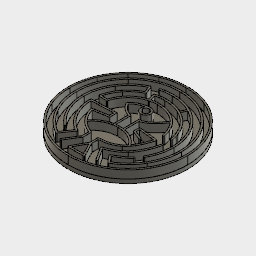
Maze 7_5 in (Autodesk Fusion 360 design; units mm, degrees)
Autodesk Fusion 360 part; units mm, degrees
sketch "Sketch5" plane through (0, 0, 0) normal (0, 1, 0) x (1, 0, 0)
  spline S0 degree 3 poles (-4.5755, 97.8232) (-27.1672, 97.8232) (-48.3865, 89.0258) (-64.3626, 73.0497) knots 0 0 0 0 1 1 1 1
  spline S1 degree 3 poles (-64.3626, 73.0497) (-80.3387, 57.0736) (-89.1009, 35.8895) (-89.1009, 13.2978) knots 0 0 0 0 1 1 1 1
  spline S2 degree 3 poles (-89.1009, 13.2978) (-89.1009, -1.7986) (-85.0541, -16.6134) (-77.4531, -29.5631) knots 0 0 0 0 1 1 1 1
  spline S3 degree 3 poles (-77.4531, -29.5631) (-70.0633, -42.1258) (-59.4713, -52.6123) (-46.8382, -59.9317) knots 0 0 0 0 1 1 1 1
  spline S4 degree 3 poles (-46.8382, -59.9317) (-46.2048, -60.2836) (-45.3954, -60.1077) (-44.9731, -59.5095) knots 0 0 0 0 1 1 1 1
  line L0 (-44.9731, -59.5095) -> (-31.9178, -40.9997)
  spline S5 degree 3 poles (-31.9178, -40.9997) (-31.4604, -40.3663) (-31.6363, -39.4866) (-32.2697, -39.0291) knots 0 0 0 0 1 1 1 1
  spline S6 degree 3 poles (-32.2697, -39.0291) (-32.3049, -38.9939) (-32.3753, -38.9939) (-32.4105, -38.9587) knots 0 0 0 0 1 1 1 1
  spline S7 degree 3 poles (-32.4105, -38.9587) (-50.2868, -29.0705) (-61.9345, -9.1884) (-62.3568, 11.9254) knots 0 0 0 0 1 1 1 1
  line L1 (-62.3568, 11.9254) -> (-27.8007, 13.2274)
  line L2 (-27.8007, 13.2274) -> (-27.8007, 6.3654)
  line L3 (-27.8007, 6.3654) -> (-50.7091, 2.389)
  spline S8 degree 3 poles (-50.7091, 2.389) (-51.5184, 2.2482) (-52.0463, 1.4037) (-51.8351, 0.6295) knots 0 0 0 0 1 1 1 1
  spline S9 degree 3 poles (-51.8351, 0.6295) (-47.7179, -14.7835) (-36.3869, -27.1351) (-21.4665, -32.6246) knots 0 0 0 0 1 1 1 1
  line L4 (-21.4665, -32.6246) -> (-21.4665, -43.6742)
  line L5 (-21.4665, -43.6742) -> (-34.2755, -64.0841)
  spline S10 degree 3 poles (-34.2755, -64.0841) (-34.6978, -64.7527) (-34.4867, -65.5973) (-33.8181, -66.0195) knots 0 0 0 0 1 1 1 1
  spline S11 degree 3 poles (-33.8181, -66.0195) (-33.5717, -66.1603) (-33.3254, -66.2307) (-33.0791, -66.2307) knots 0 0 0 0 1 1 1 1
  spline S12 degree 3 poles (-33.0791, -66.2307) (-32.6216, -66.2307) (-32.1642, -65.9843) (-31.8826, -65.5621) knots 0 0 0 0 1 1 1 1
  line L6 (-31.8826, -65.5621) -> (-18.6514, -44.4483)
  line L7 (-18.6514, -44.4483) -> (-18.6514, -31.6041)
  spline S13 degree 3 poles (-18.6514, -31.6041) (-18.6514, -31.0059) (-19.0384, -30.478) (-19.6015, -30.2669) knots 0 0 0 0 1 1 1 1
  spline S14 degree 3 poles (-19.6015, -30.2669) (-26.3227, -27.9444) (-32.2697, -24.1791) (-37.1611, -19.323) knots 0 0 0 0 1 1 1 1
  spline S15 degree 3 poles (-37.1611, -19.323) (-29.3842, -9.2235) (-17.279, -3.2061) (-4.5756, -3.2061) knots 0 0 0 0 1 1 1 1
  spline S16 degree 3 poles (-4.5756, -3.2061) (9.1484, -3.2061) (20.6906, -8.8717) (28.0804, -19.2526) knots 0 0 0 0 1 1 1 1
  spline S17 degree 3 poles (28.0804, -19.2526) (26.6024, -21.0472) (25.0541, -22.5604) (23.5057, -23.792) knots 0 0 0 0 1 1 1 1
  spline S18 degree 3 poles (23.5057, -23.792) (16.0104, -29.7743) (6.5796, -32.8006) (-4.5755, -32.8006) knots 0 0 0 0 1 1 1 1
  spline S19 degree 3 poles (-4.5755, -32.8006) (-5.3497, -32.8006) (-5.9831, -33.434) (-5.9831, -34.2082) knots 0 0 0 0 1 1 1 1
  line L8 (-5.9831, -34.2082) -> (-5.9831, -45.8207)
  line L9 (-5.9831, -45.8207) -> (-18.1235, -67.9198)
  spline S20 degree 3 poles (-18.1235, -67.9198) (-18.3698, -68.342) (-18.3698, -68.8699) (-18.0883, -69.3274) knots 0 0 0 0 1 1 1 1
  spline S21 degree 3 poles (-18.0883, -69.3274) (-17.842, -69.7496) (-17.3845, -70.0311) (-16.8919, -70.0311) knots 0 0 0 0 1 1 1 1
  line L10 (-16.8919, -70.0311) -> (7.0371, -70.0311)
  spline S22 degree 3 poles (7.0371, -70.0311) (7.5297, -70.0311) (7.9872, -69.7848) (8.2335, -69.3625) knots 0 0 0 0 1 1 1 1
  spline S23 degree 3 poles (8.2335, -69.3625) (8.4798, -68.9403) (8.515, -68.4124) (8.2687, -67.9901) knots 0 0 0 0 1 1 1 1
  line L11 (8.2687, -67.9901) -> (-3.1679, -45.8207)
  line L12 (-3.1679, -45.8207) -> (-3.1679, -35.5806)
  spline S24 degree 3 poles (-3.1679, -35.5806) (8.0224, -35.3342) (17.5587, -32.132) (25.2653, -26.009) knots 0 0 0 0 1 1 1 1
  spline S25 degree 3 poles (25.2653, -26.009) (33.2885, -19.6397) (40.7487, -5.9861) (44.3028, 8.7583) knots 0 0 0 0 1 1 1 1
  spline S26 degree 3 poles (44.3028, 8.7583) (44.4084, 9.1454) (44.3028, 9.5677) (44.0917, 9.8844) knots 0 0 0 0 1 1 1 1
  spline S27 degree 3 poles (44.0917, 9.8844) (43.8454, 10.2011) (43.4935, 10.4474) (43.1064, 10.4826) knots 0 0 0 0 1 1 1 1
  line L13 (43.1064, 10.4826) -> (14.6028, 13.6497)
  spline S28 degree 3 poles (14.6028, 13.6497) (14.2157, 13.6849) (13.7935, 13.5793) (13.5119, 13.2978) knots 0 0 0 0 1 1 1 1
  spline S29 degree 3 poles (13.5119, 13.2978) (13.2304, 13.0163) (13.0545, 12.6644) (13.0545, 12.2421) knots 0 0 0 0 1 1 1 1
  line L14 (13.0545, 12.2421) -> (13.0545, 4.4709)
  spline S30 degree 3 poles (13.0545, 4.4709) (13.0545, 3.943) (13.3712, 3.4152) (13.8638, 3.2041) knots 0 0 0 0 1 1 1 1
  line L15 (13.8638, 3.2041) -> (27.7716, -2.4085)
  spline S31 degree 3 poles (27.7716, -2.4085) (28.4754, -2.7252) (29.3199, -2.4436) (29.6366, -1.7399) knots 0 0 0 0 1 1 1 1
  spline S32 degree 3 poles (29.6366, -1.7399) (29.9533, -1.0361) (29.6718, -0.1915) (28.968, 0.1252) knots 0 0 0 0 1 1 1 1
  line L16 (28.968, 0.1252) -> (15.8345, 5.3506)
  line L17 (15.8345, 5.3506) -> (15.8345, 10.6586)
  line L18 (15.8345, 10.6586) -> (41.171, 7.8434)
  spline S33 degree 3 poles (41.171, 7.8434) (38.7077, -1.6578) (34.5905, -10.5256) (29.8751, -16.9653) knots 0 0 0 0 1 1 1 1
  spline S34 degree 3 poles (29.8751, -16.9653) (23.6114, -8.5549) (14.7436, -3.1358) (4.2219, -1.2003) knots 0 0 0 0 1 1 1 1
  line L19 (4.2219, -1.2003) -> (4.2219, 21.6377)
  spline S35 degree 3 poles (4.2219, 21.6377) (15.4474, 24.1714) (24.5967, 35.4672) (30.79, 44.5109) knots 0 0 0 0 1 1 1 1
  spline S36 degree 3 poles (30.79, 44.5109) (34.133, 40.816) (36.8074, 36.5581) (38.6373, 31.8075) knots 0 0 0 0 1 1 1 1
  spline S37 degree 3 poles (38.6373, 31.8075) (40.5023, 27.0217) (40.5023, 27.0217) (41.4876, 21.9544) knots 0 0 0 0 1 1 1 1
  line L20 (41.4876, 21.9544) -> (41.5228, 21.8137)
  spline S38 degree 3 poles (41.5228, 21.8137) (41.6636, 21.1451) (42.2266, 20.6876) (42.8952, 20.6876) knots 0 0 0 0 1 1 1 1
  spline S39 degree 3 poles (42.8952, 20.6876) (43.0008, 20.6876) (43.0712, 20.6876) (43.1767, 20.7228) knots 0 0 0 0 1 1 1 1
  spline S40 degree 3 poles (43.1767, 20.7228) (43.9509, 20.8635) (44.4436, 21.6025) (44.2676, 22.3767) knots 0 0 0 0 1 1 1 1
  line L21 (44.2676, 22.3767) -> (44.2324, 22.5174)
  spline S41 degree 3 poles (44.2324, 22.5174) (43.1767, 27.7607) (43.1416, 27.8663) (41.2413, 32.828) knots 0 0 0 0 1 1 1 1
  spline S42 degree 3 poles (41.2413, 32.828) (34.3442, 50.6691) (16.3623, 62.2113) (-4.5755, 62.2113) knots 0 0 0 0 1 1 1 1
  spline S43 degree 3 poles (-4.5755, 62.2113) (-8.4815, 62.2113) (-12.282, 61.7538) (-15.9417, 60.8741) knots 0 0 0 0 1 1 1 1
  line L22 (-15.9417, 60.8741) -> (-18.3346, 69.39)
  spline S44 degree 3 poles (-18.3346, 69.39) (-13.7952, 70.5161) (-9.115, 71.0791) (-4.3996, 71.0791) knots 0 0 0 0 1 1 1 1
  spline S45 degree 3 poles (-4.3996, 71.0791) (4.5034, 71.0791) (13.0193, 69.214) (20.9018, 65.5895) knots 0 0 0 0 1 1 1 1
  spline S46 degree 3 poles (20.9018, 65.5895) (34.9424, 59.0794) (45.3937, 47.6428) (50.3906, 33.3207) knots 0 0 0 0 1 1 1 1
  spline S47 degree 3 poles (50.3906, 33.3207) (50.9537, 31.7019) (51.3407, 30.6463) (51.6223, 29.8721) knots 0 0 0 0 1 1 1 1
  spline S48 degree 3 poles (51.6223, 29.8721) (52.3964, 27.7959) (52.502, 27.5496) (53.5225, 22.5175) knots 0 0 0 0 1 1 1 1
  spline S49 degree 3 poles (53.5225, 22.5175) (53.6633, 21.8489) (54.2263, 21.3914) (54.8949, 21.3914) knots 0 0 0 0 1 1 1 1
  spline S50 degree 3 poles (54.8949, 21.3914) (55.0005, 21.3914) (55.0709, 21.3914) (55.1764, 21.4266) knots 0 0 0 0 1 1 1 1
  spline S51 degree 3 poles (55.1764, 21.4266) (55.9506, 21.5673) (56.4432, 22.3063) (56.2673, 23.0805) knots 0 0 0 0 1 1 1 1
  spline S52 degree 3 poles (56.2673, 23.0805) (55.2116, 28.3238) (55.0708, 28.7108) (54.2615, 30.8926) knots 0 0 0 0 1 1 1 1
  spline S53 degree 3 poles (54.2615, 30.8926) (53.9448, 31.702) (53.5929, 32.6873) (53.0298, 34.2708) knots 0 0 0 0 1 1 1 1
  spline S54 degree 3 poles (53.0298, 34.2708) (48.1737, 48.2762) (38.2854, 59.6777) (25.0541, 66.7156) knots 0 0 0 0 1 1 1 1
  line L23 (25.0541, 66.7156) -> (28.7842, 74.7036)
  spline S55 degree 3 poles (28.7842, 74.7036) (51.3407, 62.4225) (65.2758, 39.0566) (65.2758, 13.333) knots 0 0 0 0 1 1 1 1
  spline S56 degree 3 poles (65.2758, 13.333) (65.2758, 0.9463) (62.0032, -11.1941) (55.7746, -21.8214) knots 0 0 0 0 1 1 1 1
  spline S57 degree 3 poles (55.7746, -21.8214) (55.3876, -22.49) (55.5987, -23.3697) (56.2673, -23.7568) knots 0 0 0 0 1 1 1 1
  spline S58 degree 3 poles (56.2673, -23.7568) (56.4784, -23.8976) (56.7248, -23.9328) (56.9711, -23.9328) knots 0 0 0 0 1 1 1 1
  spline S59 degree 3 poles (56.9711, -23.9328) (57.4637, -23.9328) (57.9212, -23.6864) (58.2027, -23.229) knots 0 0 0 0 1 1 1 1
  spline S60 degree 3 poles (58.2027, -23.229) (64.6424, -12.1794) (68.0558, 0.4888) (68.0558, 13.3682) knots 0 0 0 0 1 1 1 1
  spline S61 degree 3 poles (68.0558, 13.3682) (68.0558, 40.6401) (52.9947, 65.3784) (28.749, 77.9411) knots 0 0 0 0 1 1 1 1
  spline S62 degree 3 poles (28.749, 77.9411) (18.5089, 83.2547) (6.9667, 86.0347) (-4.6107, 86.0347) knots 0 0 0 0 1 1 1 1
  spline S63 degree 3 poles (-4.6107, 86.0347) (-10.98, 86.0347) (-17.3141, 85.1901) (-23.4371, 83.5714) knots 0 0 0 0 1 1 1 1
  spline S64 degree 3 poles (-23.4371, 83.5714) (-24.1761, 83.3603) (-24.6336, 82.5861) (-24.4224, 81.8471) knots 0 0 0 0 1 1 1 1
  spline S65 degree 3 poles (-24.4224, 81.8471) (-24.2113, 81.1081) (-23.4371, 80.6507) (-22.6981, 80.8618) knots 0 0 0 0 1 1 1 1
  spline S66 degree 3 poles (-22.6981, 80.8618) (-16.8215, 82.4453) (-10.7337, 83.2195) (-4.6107, 83.2195) knots 0 0 0 0 1 1 1 1
  spline S67 degree 3 poles (-4.6107, 83.2195) (6.2277, 83.2195) (16.6086, 80.7914) (26.2506, 76.0409) knots 0 0 0 0 1 1 1 1
  line L24 (26.2506, 76.0409) -> (22.5205, 67.9472)
  spline S68 degree 3 poles (22.5205, 67.9472) (22.3797, 68.0176) (22.239, 68.088) (22.063, 68.1583) knots 0 0 0 0 1 1 1 1
  spline S69 degree 3 poles (22.063, 68.1583) (13.8286, 71.994) (4.8905, 73.9294) (-4.4347, 73.9294) knots 0 0 0 0 1 1 1 1
  spline S70 degree 3 poles (-4.4347, 73.9294) (-9.8891, 73.9294) (-15.2731, 73.2256) (-20.4812, 71.7829) knots 0 0 0 0 1 1 1 1
  spline S71 degree 3 poles (-20.4812, 71.7829) (-21.2202, 71.5717) (-21.6776, 70.7976) (-21.4665, 70.0586) knots 0 0 0 0 1 1 1 1
  spline S72 degree 3 poles (-21.4665, 70.0586) (-21.4665, 70.0234) (-21.4665, 70.0234) (-21.4313, 69.9882) knots 0 0 0 0 1 1 1 1
  spline S73 degree 3 poles (-21.4313, 69.9882) (-21.4313, 69.953) (-21.4313, 69.953) (-21.4313, 69.9178) knots 0 0 0 0 1 1 1 1
  line L25 (-21.4313, 69.9178) -> (-18.6865, 60.1351)
  spline S74 degree 3 poles (-18.6865, 60.1351) (-34.2403, 55.4549) (-46.8382, 43.1737) (-51.5536, 27.0569) knots 0 0 0 0 1 1 1 1
  line L26 (-51.5536, 27.0569) -> (-60.5973, 27.5496)
  spline S75 degree 3 poles (-60.5973, 27.5496) (-58.5915, 35.432) (-54.8614, 42.9274) (-49.7589, 49.2967) knots 0 0 0 0 1 1 1 1
  spline S76 degree 3 poles (-49.7589, 49.2967) (-44.3749, 56.0179) (-37.4426, 61.5779) (-29.7009, 65.3432) knots 0 0 0 0 1 1 1 1
  spline S77 degree 3 poles (-29.7009, 65.3432) (-29.0322, 65.6599) (-28.7156, 66.434) (-28.9971, 67.1026) knots 0 0 0 0 1 1 1 1
  line L27 (-28.9971, 67.1026) -> (-33.3958, 78.3985)
  spline S78 degree 3 poles (-33.3958, 78.3985) (-33.5366, 78.7504) (-33.8181, 79.0319) (-34.17, 79.2079) knots 0 0 0 0 1 1 1 1
  spline S79 degree 3 poles (-34.17, 79.2079) (-34.5219, 79.3486) (-34.9441, 79.3486) (-35.296, 79.1727) knots 0 0 0 0 1 1 1 1
  spline S80 degree 3 poles (-35.296, 79.1727) (-47.6476, 73.4016) (-58.0989, 64.2875) (-65.5591, 52.8157) knots 0 0 0 0 1 1 1 1
  spline S81 degree 3 poles (-65.5591, 52.8157) (-73.1952, 41.0624) (-77.242, 27.3736) (-77.242, 13.2978) knots 0 0 0 0 1 1 1 1
  spline S82 degree 3 poles (-77.242, 13.2978) (-77.242, -8.2382) (-67.776, -28.5074) (-51.2721, -42.3721) knots 0 0 0 0 1 1 1 1
  spline S83 degree 3 poles (-51.2721, -42.3721) (-51.0258, -42.5833) (-50.6739, -42.6889) (-50.3572, -42.6889) knots 0 0 0 0 1 1 1 1
  spline S84 degree 3 poles (-50.3572, -42.6889) (-49.9701, -42.6889) (-49.5478, -42.5129) (-49.2663, -42.1962) knots 0 0 0 0 1 1 1 1
  spline S85 degree 3 poles (-49.2663, -42.1962) (-48.7736, -41.598) (-48.844, -40.7182) (-49.4422, -40.2256) knots 0 0 0 0 1 1 1 1
  spline S86 degree 3 poles (-49.4422, -40.2256) (-65.3128, -26.8887) (-74.3917, -7.3937) (-74.3917, 13.2978) knots 0 0 0 0 1 1 1 1
  spline S87 degree 3 poles (-74.3917, 13.2978) (-74.3917, 26.8458) (-70.5208, 39.9715) (-63.1662, 51.3025) knots 0 0 0 0 1 1 1 1
  spline S88 degree 3 poles (-63.1662, 51.3025) (-56.269, 61.8946) (-46.6975, 70.4105) (-35.4368, 75.9704) knots 0 0 0 0 1 1 1 1
  line L28 (-35.4368, 75.9704) -> (-32.0234, 67.2786)
  spline S89 degree 3 poles (-32.0234, 67.2786) (-39.6595, 63.3726) (-46.5215, 57.7774) (-51.8703, 51.0562) knots 0 0 0 0 1 1 1 1
  spline S90 degree 3 poles (-51.8703, 51.0562) (-57.571, 43.9127) (-61.653, 35.432) (-63.6588, 26.5291) knots 0 0 0 0 1 1 1 1
  spline S91 degree 3 poles (-63.6588, 26.5291) (-63.6588, 26.4587) (-63.694, 26.3883) (-63.694, 26.2827) knots 0 0 0 0 1 1 1 1
  spline S92 degree 3 poles (-63.694, 26.2827) (-63.7292, 25.5086) (-63.131, 24.84) (-62.3568, 24.8048) knots 0 0 0 0 1 1 1 1
  line L29 (-62.3568, 24.8048) -> (-50.4979, 24.1714)
  spline S93 degree 3 poles (-50.4979, 24.1714) (-50.0053, 24.1362) (-49.5478, 24.3825) (-49.2663, 24.8048) knots 0 0 0 0 1 1 1 1
  spline S94 degree 3 poles (-49.2663, 24.8048) (-49.1607, 24.9455) (-49.0904, 25.0863) (-49.0552, 25.2622) knots 0 0 0 0 1 1 1 1
  spline S95 degree 3 poles (-49.0552, 25.2622) (-44.7972, 41.2031) (-32.4105, 53.3083) (-17.0678, 57.6366) knots 0 0 0 0 1 1 1 1
  spline S96 degree 3 poles (-17.0678, 57.6366) (-16.9974, 57.6366) (-16.9271, 57.6014) (-16.8567, 57.6014) knots 0 0 0 0 1 1 1 1
  spline S97 degree 3 poles (-16.8567, 57.6014) (-16.7159, 57.6014) (-16.6104, 57.6014) (-16.4696, 57.6718) knots 0 0 0 0 1 1 1 1
  spline S98 degree 3 poles (-16.4696, 57.6718) (-16.2585, 57.7422) (-16.1177, 57.8126) (-15.9418, 57.9533) knots 0 0 0 0 1 1 1 1
  spline S99 degree 3 poles (-15.9418, 57.9533) (-12.2821, 58.9035) (-8.4464, 59.3961) (-4.5052, 59.3961) knots 0 0 0 0 1 1 1 1
  spline S100 degree 3 poles (-4.5052, 59.3961) (8.5854, 59.3961) (20.4443, 54.6455) (28.8546, 46.5519) knots 0 0 0 0 1 1 1 1
  spline S101 degree 3 poles (28.8546, 46.5519) (22.7316, 37.5434) (13.5471, 26.0012) (2.6383, 24.1713) knots 0 0 0 0 1 1 1 1
  spline S102 degree 3 poles (2.6383, 24.1713) (1.9697, 24.0658) (1.4771, 23.4676) (1.4771, 22.799) knots 0 0 0 0 1 1 1 1
  line L30 (1.4771, 22.799) -> (1.4771, -0.7781)
  spline S103 degree 3 poles (1.4771, -0.7781) (-0.4584, -0.5317) (-2.4642, -0.4262) (-4.5052, -0.4262) knots 0 0 0 0 1 1 1 1
  spline S104 degree 3 poles (-4.5052, -0.4262) (-6.4054, -0.4262) (-8.2705, -0.5669) (-10.1355, -0.8133) knots 0 0 0 0 1 1 1 1
  line L31 (-10.1355, -0.8133) -> (-10.1355, 22.7286)
  spline S105 degree 3 poles (-10.1355, 22.7286) (-10.1003, 23.3972) (-10.5578, 24.0306) (-11.2264, 24.1714) knots 0 0 0 0 1 1 1 1
  spline S106 degree 3 poles (-11.2264, 24.1714) (-18.1939, 25.6845) (-23.8242, 29.9776) (-28.4341, 37.2619) knots 0 0 0 0 1 1 1 1
  spline S107 degree 3 poles (-28.4341, 37.2619) (-23.6835, 41.9773) (-17.8068, 45.1443) (-11.3671, 46.4464) knots 0 0 0 0 1 1 1 1
  spline S108 degree 3 poles (-11.3671, 46.4464) (-12.3524, 45.074) (-12.9507, 43.4201) (-12.9507, 41.5902) knots 0 0 0 0 1 1 1 1
  spline S109 degree 3 poles (-12.9507, 41.5902) (-12.9507, 37.0156) (-9.2558, 33.3207) (-4.6811, 33.3207) knots 0 0 0 0 1 1 1 1
  spline S110 degree 3 poles (-4.6811, 33.3207) (-0.1065, 33.3207) (3.5884, 37.0156) (3.5884, 41.5902) knots 0 0 0 0 1 1 1 1
  spline S111 degree 3 poles (3.5884, 41.5902) (3.5884, 46.0945) (-0.0361, 49.7542) (-4.5052, 49.8598) knots 0 0 0 0 1 1 1 1
  line L32 (-4.5052, 49.8598) -> (-4.5052, 49.9653)
  spline S112 degree 3 poles (-4.5052, 49.9653) (-14.675, 49.9653) (-24.141, 45.8833) (-31.1437, 38.5287) knots 0 0 0 0 1 1 1 1
  spline S113 degree 3 poles (-31.1437, 38.5287) (-31.1789, 38.4935) (-31.1789, 38.4935) (-31.2141, 38.4583) knots 0 0 0 0 1 1 1 1
  spline S114 degree 3 poles (-31.2141, 38.4583) (-31.6363, 38.0009) (-31.7419, 37.3323) (-31.39, 36.7692) knots 0 0 0 0 1 1 1 1
  spline S115 degree 3 poles (-31.39, 36.7692) (-26.4987, 28.6404) (-20.4461, 23.7139) (-12.9155, 21.7433) knots 0 0 0 0 1 1 1 1
  line L33 (-12.9155, 21.7433) -> (-12.9155, -1.2707)
  spline S116 degree 3 poles (-12.9155, -1.2707) (-23.1205, -3.3117) (-32.4457, -8.942) (-38.991, -17.282) knots 0 0 0 0 1 1 1 1
  spline S117 degree 3 poles (-38.991, -17.282) (-43.3193, -12.3906) (-46.6271, -6.5491) (-48.5625, -0.1095) knots 0 0 0 0 1 1 1 1
  line L34 (-48.5625, -0.1095) -> (-24.8447, 4.0429)
  line L35 (-24.8447, 4.0429) -> (-24.8447, 16.1833)
  line L36 (-24.8447, 16.1833) -> (-63.7644, 14.7054)
  spline S118 degree 3 poles (-63.7644, 14.7054) (-64.5386, 14.6702) (-65.1368, 14.0368) (-65.1016, 13.2626) knots 0 0 0 0 1 1 1 1
  spline S119 degree 3 poles (-65.1016, 13.2626) (-65.1016, 13.2274) (-65.1016, 13.1922) (-65.1016, 13.157) knots 0 0 0 0 1 1 1 1
  line L37 (-65.1016, 13.157) -> (-65.2072, 13.157)
  spline S120 degree 3 poles (-65.2072, 13.157) (-65.2072, -8.8716) (-53.4538, -29.8094) (-35.1201, -40.6126) knots 0 0 0 0 1 1 1 1
  line L38 (-35.1201, -40.6126) -> (-46.5567, -56.7998)
  spline S121 degree 3 poles (-46.5567, -56.7998) (-58.2748, -49.7619) (-68.0927, -39.8737) (-75.025, -28.0852) knots 0 0 0 0 1 1 1 1
  spline S122 degree 3 poles (-75.025, -28.0852) (-82.3797, -15.5929) (-86.2857, -1.2355) (-86.2857, 13.3682) knots 0 0 0 0 1 1 1 1
  spline S123 degree 3 poles (-86.2857, 13.3682) (-86.2857, 35.1857) (-77.7698, 55.7364) (-62.3568, 71.1495) knots 0 0 0 0 1 1 1 1
  spline S124 degree 3 poles (-62.3568, 71.1495) (-46.9438, 86.5625) (-26.393, 95.0784) (-4.5755, 95.0784) knots 0 0 0 0 1 1 1 1
  spline S125 degree 3 poles (-4.5755, 95.0784) (17.242, 95.0784) (37.7928, 86.5625) (53.2058, 71.1495) knots 0 0 0 0 1 1 1 1
  spline S126 degree 3 poles (53.2058, 71.1495) (68.6188, 55.7364) (77.1347, 35.1857) (77.1347, 13.3682) knots 0 0 0 0 1 1 1 1
  spline S127 degree 3 poles (77.1347, 13.3682) (77.1347, -1.2355) (73.2287, -15.5577) (65.874, -28.0852) knots 0 0 0 0 1 1 1 1
  spline S128 degree 3 poles (65.874, -28.0852) (58.9065, -39.9088) (49.0534, -49.7971) (37.3001, -56.8351) knots 0 0 0 0 1 1 1 1
  line L39 (37.3001, -56.8351) -> (30.2974, -48.6007)
  spline S129 degree 3 poles (30.2974, -48.6007) (37.3705, -44.5187) (45.9567, -39.4514) (51.0592, -33.3636) knots 0 0 0 0 1 1 1 1
  spline S130 degree 3 poles (51.0592, -33.3636) (51.5519, -32.7654) (51.4815, -31.8856) (50.8833, -31.393) knots 0 0 0 0 1 1 1 1
  spline S131 degree 3 poles (50.8833, -31.393) (50.285, -30.9003) (49.4053, -30.9707) (48.9127, -31.5689) knots 0 0 0 0 1 1 1 1
  spline S132 degree 3 poles (48.9127, -31.5689) (43.9509, -37.4808) (35.2239, -42.5129) (28.2564, -46.5597) knots 0 0 0 0 1 1 1 1
  line L40 (28.2564, -46.5597) -> (27.447, -47.0171)
  spline S133 degree 3 poles (27.447, -47.0171) (27.0951, -47.2283) (26.8488, -47.5802) (26.7784, -48.0025) knots 0 0 0 0 1 1 1 1
  spline S134 degree 3 poles (26.7784, -48.0025) (26.708, -48.4247) (26.8136, -48.847) (27.0951, -49.1637) knots 0 0 0 0 1 1 1 1
  line L41 (27.0951, -49.1637) -> (35.9277, -59.5798)
  spline S135 degree 3 poles (35.9277, -59.5798) (36.2092, -59.8965) (36.5963, -60.0725) (37.0186, -60.0725) knots 0 0 0 0 1 1 1 1
  spline S136 degree 3 poles (37.0186, -60.0725) (37.2649, -60.0725) (37.5112, -60.0021) (37.7224, -59.8965) knots 0 0 0 0 1 1 1 1
  spline S137 degree 3 poles (37.7224, -59.8965) (50.3554, -52.6123) (60.9123, -42.0906) (68.3373, -29.5279) knots 0 0 0 0 1 1 1 1
  spline S138 degree 3 poles (68.3373, -29.5279) (75.9734, -16.5782) (79.985, -1.7633) (79.985, 13.333) knots 0 0 0 0 1 1 1 1
  spline S139 degree 3 poles (79.985, 13.333) (79.985, 35.9247) (71.1876, 57.144) (55.2116, 73.1201) knots 0 0 0 0 1 1 1 1
  spline S140 degree 3 poles (55.2116, 73.1201) (39.2355, 89.061) (18.0162, 97.8232) (-4.5755, 97.8232) knots 0 0 0 0 1 1 1 1
  line L42 (-14.5342, -67.1808) -> (-4.6107, -49.1637)
  line L43 (-4.6107, -49.1637) -> (4.7497, -67.1808)
  line L44 (4.7497, -67.1808) -> (-14.5342, -67.1808)
  spline S141 degree 3 poles (0.7029, 41.6254) (0.7029, 38.6343) (-1.7603, 36.171) (-4.7515, 36.171) knots 0 0 0 0 1 1 1 1
  spline S142 degree 3 poles (-4.7515, 36.171) (-7.7426, 36.171) (-10.2058, 38.6343) (-10.2058, 41.6254) knots 0 0 0 0 1 1 1 1
  spline S143 degree 3 poles (-10.2058, 41.6254) (-10.2058, 44.6165) (-7.7426, 47.0798) (-4.7515, 47.0798) knots 0 0 0 0 1 1 1 1
  spline S144 degree 3 poles (-4.7515, 47.0798) (-1.7603, 47.0798) (0.7029, 44.6165) (0.7029, 41.6254) knots 0 0 0 0 1 1 1 1
  spline S145 degree 3 poles (13.0193, -45.1169) (22.3797, -42.3018) (31.1067, -36.9529) (38.3206, -29.5983) knots 0 0 0 0 1 1 1 1
  spline S146 degree 3 poles (38.3206, -29.5983) (47.2236, -20.5194) (53.8744, -3.8747) (56.2673, 7.7378) knots 0 0 0 0 1 1 1 1
  spline S147 degree 3 poles (56.2673, 7.7378) (56.4081, 8.512) (55.9506, 9.251) (55.1764, 9.3917) knots 0 0 0 0 1 1 1 1
  spline S148 degree 3 poles (55.1764, 9.3917) (54.4022, 9.5325) (53.6633, 9.075) (53.5225, 8.3009) knots 0 0 0 0 1 1 1 1
  spline S149 degree 3 poles (53.5225, 8.3009) (50.2147, -7.7104) (42.297, -21.5751) (36.35, -27.6277) knots 0 0 0 0 1 1 1 1
  spline S150 degree 3 poles (36.35, -27.6277) (29.0306, -35.0879) (20.0924, -40.3663) (10.5208, -42.9352) knots 0 0 0 0 1 1 1 1
  spline S151 degree 3 poles (10.5208, -42.9352) (9.7819, -43.1463) (9.3244, -43.9205) (9.5355, -44.6595) knots 0 0 0 0 1 1 1 1
  spline S152 degree 3 poles (9.5355, -44.6595) (9.5355, -44.6946) (9.5355, -44.6946) (9.5707, -44.7298) knots 0 0 0 0 1 1 1 1
  spline S153 degree 3 poles (9.5707, -44.7298) (9.6059, -44.9058) (9.6763, -45.0466) (9.7467, -45.1873) knots 0 0 0 0 1 1 1 1
  line L45 (9.7467, -45.1873) -> (22.7668, -65.5973)
  spline S154 degree 3 poles (22.7668, -65.5973) (23.0483, -66.0195) (23.5058, -66.2307) (23.9633, -66.2307) knots 0 0 0 0 1 1 1 1
  spline S155 degree 3 poles (23.9633, -66.2307) (24.2096, -66.2307) (24.4911, -66.1603) (24.7022, -66.0195) knots 0 0 0 0 1 1 1 1
  spline S156 degree 3 poles (24.7022, -66.0195) (25.3708, -65.5973) (25.5468, -64.7175) (25.1245, -64.0841) knots 0 0 0 0 1 1 1 1
  line L46 (25.1245, -64.0841) -> (13.0193, -45.1169)
  spline S157 degree 3 poles (-4.9274, 108.3097) (-57.3951, 108.3097) (-99.9393, 65.7655) (-99.9393, 13.2978) knots 0 0 0 0 1 1 1 1
  spline S158 degree 3 poles (-99.9393, 13.2978) (-99.9393, -39.1699) (-57.3951, -81.7141) (-4.9274, -81.7141) knots 0 0 0 0 1 1 1 1
  spline S159 degree 3 poles (-4.9274, -81.7141) (47.5403, -81.7141) (90.0845, -39.1699) (90.0845, 13.2978) knots 0 0 0 0 1 1 1 1
  spline S160 degree 3 poles (90.0845, 13.2978) (90.0845, 65.7654) (47.5403, 108.3097) (-4.9274, 108.3097) knots 0 0 0 0 1 1 1 1
  spline S161 degree 3 poles (60.2789, -51.9085) (51.7982, -60.3892) (41.9451, -67.04) (30.966, -71.6851) knots 0 0 0 0 1 1 1 1
  spline S162 degree 3 poles (30.966, -71.6851) (19.5997, -76.506) (7.5297, -78.9341) (-4.9274, -78.9341) knots 0 0 0 0 1 1 1 1
  spline S163 degree 3 poles (-4.9274, -78.9341) (-17.3845, -78.9341) (-29.4545, -76.506) (-40.8208, -71.6851) knots 0 0 0 0 1 1 1 1
  spline S164 degree 3 poles (-40.8208, -71.6851) (-51.7999, -67.04) (-61.653, -60.3892) (-70.1337, -51.9085) knots 0 0 0 0 1 1 1 1
  spline S165 degree 3 poles (-70.1337, -51.9085) (-78.6144, -43.4278) (-85.2652, -33.5747) (-89.9102, -22.5956) knots 0 0 0 0 1 1 1 1
  spline S166 degree 3 poles (-89.9102, -22.5956) (-94.7312, -11.2294) (-97.1593, 0.8407) (-97.1593, 13.2978) knots 0 0 0 0 1 1 1 1
  spline S167 degree 3 poles (-97.1593, 13.2978) (-97.1593, 25.7549) (-94.7312, 37.8249) (-89.9102, 49.1912) knots 0 0 0 0 1 1 1 1
  spline S168 degree 3 poles (-89.9102, 49.1912) (-85.2652, 60.1703) (-78.6144, 70.0234) (-70.1337, 78.5041) knots 0 0 0 0 1 1 1 1
  spline S169 degree 3 poles (-70.1337, 78.5041) (-61.653, 86.9848) (-51.7999, 93.6356) (-40.8208, 98.2806) knots 0 0 0 0 1 1 1 1
  spline S170 degree 3 poles (-40.8208, 98.2806) (-29.4545, 103.1016) (-17.3845, 105.5297) (-4.9274, 105.5297) knots 0 0 0 0 1 1 1 1
  spline S171 degree 3 poles (-4.9274, 105.5297) (7.5297, 105.5297) (19.5997, 103.1016) (30.966, 98.2806) knots 0 0 0 0 1 1 1 1
  spline S172 degree 3 poles (30.966, 98.2806) (41.9451, 93.6356) (51.7982, 86.9848) (60.2789, 78.5041) knots 0 0 0 0 1 1 1 1
  spline S173 degree 3 poles (60.2789, 78.5041) (68.7596, 70.0234) (75.4104, 60.1703) (80.0554, 49.1912) knots 0 0 0 0 1 1 1 1
  spline S174 degree 3 poles (80.0554, 49.1912) (84.8764, 37.8249) (87.3045, 25.7549) (87.3045, 13.2978) knots 0 0 0 0 1 1 1 1
  spline S175 degree 3 poles (87.3045, 13.2978) (87.3045, 0.8407) (84.8764, -11.2294) (80.0554, -22.5956) knots 0 0 0 0 1 1 1 1
  spline S176 degree 3 poles (80.0554, -22.5956) (75.3752, -33.5747) (68.7244, -43.4278) (60.2789, -51.9085) knots 0 0 0 0 1 1 1 1
sketch "Sketch6" plane through (0, 0, 0) normal (0, 1, 0) x (1, 0, 0)
  circle A0 centre (-4.9274, 13.2978) radius 95.0119
  constraint coincident A0 origin
  constraint coincident A0
combine "Combine1" [no effect]
scale "Scale1" [no effect]
scale "Scale2" [no effect]
extrude "Extrude8" add sketch "Sketch5" along normal blind 12.7 makes body 1 at (-61.6036, 0, 46.3023) makes body 2 at (-9.754, 4.2333, -108.1891) makes body 3 at (50.521, 7.0556, 10.1087)
extrude "Extrude9" add sketch "Sketch6" against normal blind 6.35 bodies 1 2 3
move_body "MoveBody1" bodies 1 to x (1, 0, 0) y (0, 1, 0) z (0, 0, 1) at (0, 6.35, 0)
